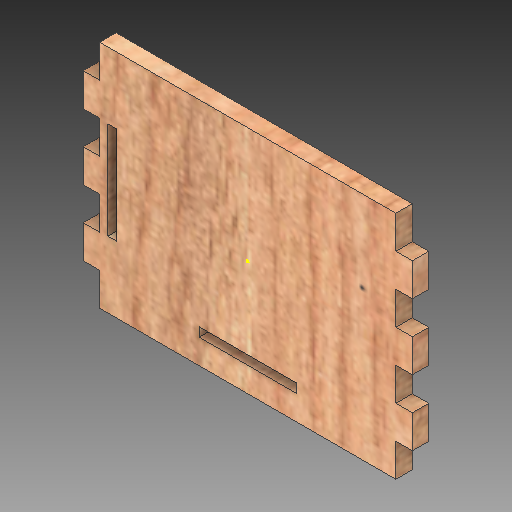
# Autodesk Inventor part: PiShelf
Saved by Autodesk Inventor 2019 (Build 230136000, 136)
## iProperties
Created: 2019-01-17
Part Number: PiShelf
Material: Wood (Birch)
Document SubType Name: Modeling
Designer: nxgam
Density: 0.55 g/cm^3
Appearance: Birch - Natural Polished
Mass: 18.3542 g
Surface Area: 157.143 cm^2
Volume: 33.3712 cm^3
Author: nxgam
Autodesk Inventor part; units mm, degrees
ref_plane "YZ Plane" through (0, 0, 0) normal (1, 0, 0) x (0, 1, 0)
ref_plane "XZ Plane" through (0, 0, 0) normal (0, 1, 0) x (-1, 0, 0)
ref_plane "XY Plane" through (0, 0, 0) normal (0, 0, 1) x (1, 0, 0)
sketch "Sketch1" plane through (0, 0, 0) normal (0, 0, 1) x (1, 0, 0)
  line L0 (-50.8, -35.56) -> (50.8, -35.56)
  line L1 (50.8, -35.56) -> (50.8, 35.56)
  line L2 (50.8, 35.56) -> (-50.8, 35.56)
  line L3 (-50.8, 35.56) -> (-50.8, -35.56)
  line L4 (-50.8, 35.56) -> (50.8, -35.56) construction
  line L5 (50.8, -35.56) -> (-50.8, -35.56) construction
  line L6 (50.8, 35.56) -> (-50.8, -35.56) construction
  point P0 (0, 0)
  point P1 (0, 0)
  dimension "d0" = 101.6
  dimension "d1" = 71.12
  constraints: 14 end point, 3 equal length, 1 coincident, 1 horizontal, 1 midpoint, 1 perpendicular
  measures "d0" distance of L2.end L1.end
  measures "d1" distance of L1.end L0.end
extrude "Extrusion1" add sketch "Sketch1" along normal blind 5.08
sketch "Sketch2" plane through (0, 0, 5.08) normal (0, 0, 1) x (1, 0, 0)
  line L0 (-43.18, 16.9024) -> (-43.18, -16.905) projected
  line L1 (-40.386, 16.9024) -> (-40.386, -16.905) projected
  line L2 (-16.9024, -27.94) -> (16.905, -27.94) projected
  line L3 (-16.9024, -25.146) -> (16.905, -25.146) projected
  line L4 (-40.386, -16.905) -> (-43.18, -16.905) projected
  line L5 (-43.18, 16.9024) -> (-40.386, 16.9024) projected
  line L6 (16.905, -25.146) -> (16.905, -27.94) projected
  line L7 (-16.9024, -27.94) -> (-16.9024, -25.146) projected
  point P0 (0, 0)
extrude "Extrusion2" cut sketch "Sketch2" against normal blind 5.08
sketch "Sketch3" plane through (0, 0, 5.08) normal (0, 0, 1) x (1, 0, 0)
  line L0 (-43.18, -16.905) -> (-43.18, 16.9024) projected
  line L1 (-40.386, 16.9024) -> (-40.386, -16.905) projected
  line L2 (16.905, -27.94) -> (-16.9024, -27.94) projected
  line L3 (-16.9024, -25.146) -> (16.905, -25.146) projected
  line L4 (50.8, -35.56) -> (50.8, 35.56) projected
  line L5 (50.8, 35.56) -> (-50.8, 35.56) projected
  line L6 (-50.8, 35.56) -> (-50.8, -35.56) projected
  line L7 (-50.8, -35.56) -> (50.8, -35.56) projected
  line L8 (50.8, -35.56) -> (50.8, 35.56) projected
  line L9 (50.8, 35.56) -> (45.72, 35.56)
  line L10 (45.72, 35.56) -> (45.72, 25.4)
  line L11 (45.72, 25.4) -> (50.8, 25.4)
  line L12 (50.8, 25.4) -> (50.8, 35.56)
  line L13 (0, 35.56) -> (0, -35.56) construction
  line L14 (45.72, 5.08) -> (50.8, 5.08)
  line L15 (45.72, 15.24) -> (45.72, 5.08)
  line L16 (50.8, 15.24) -> (45.72, 15.24)
  line L17 (50.8, 5.08) -> (50.8, 15.24)
  line L18 (45.72, -15.24) -> (50.8, -15.24)
  line L19 (45.72, -5.08) -> (45.72, -15.24)
  line L20 (50.8, -5.08) -> (45.72, -5.08)
  line L21 (50.8, -15.24) -> (50.8, -5.08)
  line L22 (45.72, -35.56) -> (50.8, -35.56)
  line L23 (45.72, -25.4) -> (45.72, -35.56)
  line L24 (50.8, -25.4) -> (45.72, -25.4)
  line L25 (50.8, -35.56) -> (50.8, -25.4)
  line L26 (-50.8, -35.56) -> (-50.8, 35.56)
  line L27 (-50.8, -35.56) -> (-50.8, 35.56)
  line L28 (-50.8, 35.56) -> (-45.72, 35.56)
  line L29 (-45.72, 35.56) -> (-45.72, 25.4)
  line L30 (-45.72, 25.4) -> (-50.8, 25.4)
  line L31 (-50.8, 25.4) -> (-50.8, 35.56)
  line L32 (-45.72, 5.08) -> (-50.8, 5.08)
  line L33 (-45.72, 15.24) -> (-45.72, 5.08)
  line L34 (-50.8, 15.24) -> (-45.72, 15.24)
  line L35 (-50.8, 5.08) -> (-50.8, 15.24)
  line L36 (-45.72, -15.24) -> (-50.8, -15.24)
  line L37 (-45.72, -5.08) -> (-45.72, -15.24)
  line L38 (-50.8, -5.08) -> (-45.72, -5.08)
  line L39 (-50.8, -15.24) -> (-50.8, -5.08)
  line L40 (-45.72, -35.56) -> (-50.8, -35.56)
  line L41 (-45.72, -25.4) -> (-45.72, -35.56)
  line L42 (-50.8, -25.4) -> (-45.72, -25.4)
  line L43 (-50.8, -35.56) -> (-50.8, -25.4)
  line L44 (-40.386, -16.905) -> (-43.18, -16.905) projected
  line L45 (-43.18, 16.9024) -> (-40.386, 16.9024) projected
  line L46 (16.905, -25.146) -> (16.905, -27.94) projected
  line L47 (-16.9024, -27.94) -> (-16.9024, -25.146) projected
  point P0 (0, 0)
  dimension "d6" = 10.16
  dimension "d7" = 5.08
  dimension "d8" = 0
  dimension "d11" = 20.32
  dimension "d16" = 20.32
  constraints: 70 end point, 18 symmetric about line, 2 midpoint, 2 parallel, 2 point on line, 1 horizontal, 1 perpendicular, 1 vertical, 24 other
  measures "d6" distance of L9.end L10.end
  measures "d7" distance of L9.start L9.end
  measures "d8" distance between parallel lines of L5 L9
  measures "d11" distance of L10.end L14.start
  measures "d16" distance between parallel lines of L7 L18
extrude "Extrusion3" cut sketch "Sketch3" against normal blind 25.4 contours L0 L45 L1 L44 | L2 L47 L3 L46 | L24 L23 L7 L41 L42 L6 L36 L37 L38 L32 L33 L34 L30 L29 L5 L10 L11 L4 L16 L15 L14 L20 L19 L18 keep common part
sketch "Sketch4" plane through (0, 0, 5.08) normal (0, 0, 1) x (1, 0, 0)
  point P0 (0, 0)
sketch "Sketch5" plane through (0, 0, 5.08) normal (0, 0, 1) x (1, 0, 0)
  line L0 (-50.8, -15.24) -> (-45.72, -15.24) projected
  line L1 (-50.8, -15.24) -> (-50.8, -25.4) projected
  line L2 (-45.72, -25.4) -> (-50.8, -25.4) projected
  line L3 (-45.72, -35.56) -> (-45.72, -25.4) projected
  line L4 (-45.72, -35.56) -> (45.72, -35.56) projected
  line L5 (45.72, -25.4) -> (45.72, -35.56) projected
  line L6 (50.8, -25.4) -> (45.72, -25.4) projected
  line L7 (50.8, -25.4) -> (50.8, -15.24) projected
  line L8 (45.72, -15.24) -> (50.8, -15.24) projected
  line L9 (45.72, -5.08) -> (45.72, -15.24) projected
  line L10 (50.8, -5.08) -> (45.72, -5.08) projected
  line L11 (50.8, -5.08) -> (50.8, 5.08) projected
  line L12 (45.72, 5.08) -> (50.8, 5.08) projected
  line L13 (45.72, 15.24) -> (45.72, 5.08) projected
  line L14 (50.8, 15.24) -> (45.72, 15.24) projected
  line L15 (50.8, 15.24) -> (50.8, 25.4) projected
  line L16 (45.72, 25.4) -> (50.8, 25.4) projected
  line L17 (45.72, 35.56) -> (45.72, 25.4) projected
  line L18 (45.72, 35.56) -> (-45.72, 35.56) projected
  line L19 (-45.72, 25.4) -> (-45.72, 35.56) projected
  line L20 (-50.8, 25.4) -> (-45.72, 25.4) projected
  line L21 (-50.8, 25.4) -> (-50.8, 15.24) projected
  line L22 (-45.72, 15.24) -> (-50.8, 15.24) projected
  line L23 (-45.72, 5.08) -> (-45.72, 15.24) projected
  line L24 (-50.8, 5.08) -> (-45.72, 5.08) projected
  line L25 (-50.8, 5.08) -> (-50.8, -5.08) projected
  line L26 (-45.72, -5.08) -> (-50.8, -5.08) projected
  line L27 (-45.72, -15.24) -> (-45.72, -5.08) projected
  line L28 (-43.18, -16.905) -> (-43.18, 16.9024) projected
  line L29 (-40.386, 16.9024) -> (-40.386, -16.905) projected
  line L30 (16.905, -27.94) -> (-16.9024, -27.94) projected
  line L31 (-16.9024, -25.146) -> (16.905, -25.146) projected
  line L32 (-40.386, 20.0774) -> (-43.18, 20.0774)
  line L33 (-43.18, 20.0774) -> (-43.18, 14.9974)
  line L34 (-43.18, 14.9974) -> (-40.386, 14.9974)
  line L35 (-40.386, 14.9974) -> (-40.386, 20.0774)
  line L36 (-43.18, -20.08) -> (-40.386, -20.08)
  line L37 (-40.386, -20.08) -> (-40.386, -15)
  line L38 (-40.386, -15) -> (-43.18, -15)
  line L39 (-43.18, -15) -> (-43.18, -20.08)
  line L40 (-20.0774, -27.94) -> (-14.9974, -27.94)
  line L41 (-14.9974, -27.94) -> (-14.9974, -25.146)
  line L42 (-14.9974, -25.146) -> (-20.0774, -25.146)
  line L43 (-20.0774, -25.146) -> (-20.0774, -27.94)
  line L44 (20.08, -25.146) -> (15, -25.146)
  line L45 (15, -25.146) -> (15, -27.94)
  line L46 (15, -27.94) -> (20.08, -27.94)
  line L47 (20.08, -27.94) -> (20.08, -25.146)
  line L48 (-40.386, -16.905) -> (-43.18, -16.905) projected
  line L49 (-43.18, 16.9024) -> (-40.386, 16.9024) projected
  line L50 (16.905, -25.146) -> (16.905, -27.94) projected
  line L51 (-16.9024, -27.94) -> (-16.9024, -25.146) projected
  point P0 (0, 0)
  dimension "d19" = 5.08
  dimension "d20" = 5.08
  dimension "d21" = 5.08
  dimension "d22" = 5.08
  constraints: 32 end point, 8 parallel, 4 horizontal, 4 perpendicular, 4 point on line
  measures "d19" distance of L33.end L32.end
  measures "d20" distance of L37.end L36.end
  measures "d21" distance of L42.end L41.end
  measures "d22" distance of L46.end L45.end
extrude "Extrusion4" add sketch "Sketch5" against normal blind 5.08 contours L48 L37 L36 L39 | L28 L38 L29 L48 | L28 L49 L29 L34 | L33 L32 L35 L49 | L50 L44 L47 L46 | L30 L45 L31 L50 | L30 L51 L31 L41 | L40 L43 L42 L51
body "Solid1"
